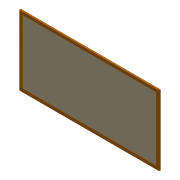
# Autodesk Inventor part: Ship area
Saved by Autodesk Inventor 2015 (Build 190159000, 159)
## iProperties
Created: 2015-03-07
Part Number: Ship area
Material: Generic
Document SubType Name: Modeling
Designer: Vukica
Density: 1 g/cm^3
Appearance: Yellow Pine - Solid Stained Light Low Gloss
Author: Vukica
Autodesk Inventor part; units mm, degrees
ref_plane "YZ Plane" through (0, 0, 0) normal (1, 0, 0) x (0, 1, 0)
ref_plane "XZ Plane" through (0, 0, 0) normal (0, 1, 0) x (-1, 0, 0)
ref_plane "XY Plane" through (0, 0, 0) normal (0, 0, 1) x (1, 0, 0)
sketch "Sketch1" plane through (0, 0, 0) normal (0, 0, 1) x (1, 0, 0)
  line L0 (0, 0) -> (1219.2, 0)
  line L1 (1219.2, 0) -> (1219.2, 609.6)
  line L2 (1219.2, 609.6) -> (0, 609.6)
  line L3 (0, 609.6) -> (0, 0)
  dimension "d0" = 1219.2
  dimension "d1" = 609.6
  constraints: 8 end point, 2 parallel, 1 horizontal, 1 perpendicular
  measures "d0" distance of L1.end L2.end
  measures "d1" distance of L2.end L0.start
extrude "Extrusion1" add sketch "Sketch1" along normal blind 12.7
sketch "Sketch2" plane through (0, 0, 12.7) normal (0, 0, 1) x (1, 0, 0)
  line L0 (0, 609.6) -> (0, 0) projected
  line L1 (1219.2, 609.6) -> (0, 609.6) projected
  line L2 (0, 0) -> (1219.2, 0) projected
  line L3 (1219.2, 0) -> (1219.2, 609.6) projected
  line L4 (1193.8, 25.4) -> (25.4, 25.4)
  line L5 (25.4, 25.4) -> (25.4, 584.2)
  line L6 (25.4, 584.2) -> (1193.8, 584.2)
  line L7 (1193.8, 584.2) -> (1193.8, 25.4)
  dimension "d4" = 25.4
  constraints: 8 end point, 3 other
  measures "d4" distance between parallel lines of L0 L5
extrude "Extrusion2" cut sketch "Sketch2" against normal blind 2.54 contours L4 L5 L6 L7
body "Solid1"
